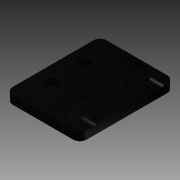
# Autodesk Inventor part: GANTRY SIDE PLATE
Saved by Autodesk Inventor 2013 (Build 170138000, 138)
## iProperties
Created: 2014-03-03
Part Number: GANTRY SIDE PLATE
Material: Generic
Document SubType Name: Modeling
Designer: employee
Density: 1 g/cm^3
Author: employee
Autodesk Inventor part; units mm, degrees
ref_plane "YZ Plane" through (0, 0, 0) normal (1, 0, 0) x (0, 1, 0)
ref_plane "XZ Plane" through (0, 0, 0) normal (0, 1, 0) x (-1, 0, 0)
ref_plane "XY Plane" through (0, 0, 0) normal (0, 0, 1) x (1, 0, 0)
sketch "Sketch1" plane through (0, 0, 0) normal (0, 0, 1) x (1, 0, 0)
  line L0 (0, 35) -> (55, 35)
  line L1 (55, -35) -> (0, -35)
  line L2 (0, -35) -> (0, 35)
  line L3 (11, 12.5) -> (11, -12.5) construction
  circle A0 centre (11, 12.5) radius 11 construction
  circle A1 centre (11, -12.5) radius 11 construction
  circle A2 centre (11, 12.5) radius 4
  circle A3 centre (11, -12.5) radius 4
  line L4 (27.1967, 8.5) -> (37.8033, 8.5) construction
  line L5 (37.8033, 8.5) -> (37.8033, -8.5) construction
  line L6 (37.8033, -8.5) -> (27.1967, -8.5) construction
  line L7 (27.1967, -8.5) -> (27.1967, 8.5) construction
  line L8 (37.8033, 8.5) -> (27.1967, 8.5)
  line L9 (27.1967, 8.5) -> (27.1967, 32.5)
  line L10 (27.1967, 32.5) -> (37.8033, 32.5)
  line L11 (37.8033, 32.5) -> (37.8033, 8.5)
  line L12 (37.8033, -8.5) -> (27.1967, -8.5)
  line L13 (27.1967, -8.5) -> (27.1967, -32.5)
  line L14 (27.1967, -32.5) -> (37.8033, -32.5)
  line L15 (37.8033, -32.5) -> (37.8033, -8.5)
  circle A4 centre (32.5, 8.5) radius 7.5 construction
  line L16 (32.5, 8.5) -> (37.8033, 3.1967) construction
  line L17 (55, 27.8284) -> (45, 27.8284)
  line L18 (45, 27.8284) -> (45, 22.1716)
  line L19 (45, 22.1716) -> (55, 22.1716)
  line L20 (55, -27.8284) -> (45, -27.8284)
  line L21 (45, -27.8284) -> (45, -22.1716)
  line L22 (45, -22.1716) -> (55, -22.1716)
  line L23 (55, -27.8284) -> (55, -35)
  line L24 (55, 35) -> (55, 27.8284)
  line L25 (55, 22.1716) -> (55, -22.1716)
  circle A5 centre (45, 25) radius 4 construction
  line L26 (45, 25) -> (42.1716, 22.1716) construction
  point P0 (0, 0)
  point P1 (0, 0)
  point P2 (11, 0)
  point P3 (27.1967, 0)
  point P4 (45, -25)
  dimension "d7" = 15
  dimension "d16" = 8
  dimension "d0" = 70
  dimension "d2" = 11
  dimension "d3" = 25
  dimension "d4" = 8
  dimension "d5" = 24
  dimension "d6" = 45
  dimension "d9" = 2.5
  dimension "d11" = 22.5
  dimension "d12" = 55
  dimension "d13" = 10
  dimension "d15" = 45
  dimension "d17" = 10
  constraints: 54 end point, 13 parallel, 8 perpendicular, 6 coincident, 6 equal length, 6 horizontal, 6 midpoint, 4 centre point, 3 horizontal alignment, 2 equal radius, 1 point on line, 1 tangent, 6 other
  measures "d0" distance of L1.end L0.start
  measures "d2" distance between parallel lines of L3 L2
  measures "d3" distance of L3.start L3.end
  measures "d4" diameter of A2
  measures "d5" distance of L4.start L9.end
  measures "d6" angle of L8 L16
  measures "d9" distance between parallel lines of L0 L10
  measures "d11" distance from line of L25 L16.start
  measures "d12" distance of L1.start L1.end
  measures "d13" distance from line of L0 point (45, 25)
  measures "d15" angle of L18 L26
  measures "d17" distance of L18.end L19.end
extrude "Extrusion1" add sketch "Sketch1" along normal blind 6.477
sketch "Sketch2" plane through (0, 0, 6.477) normal (0, 0, 1) x (1, 0, 0)
  line L0 (27.1967, 8.5) -> (27.1967, 32.5) projected
  line L1 (27.1967, 32.5) -> (37.8033, 32.5) projected
  line L2 (45, 22.1716) -> (45, 27.8284) projected
  line L3 (45, 27.8284) -> (55, 27.8284) projected
  line L4 (25, 25.5) -> (40, 25.5) construction
  line L5 (40, 25.5) -> (40, 15.5) construction
  line L6 (40, 15.5) -> (25, 15.5) construction
  line L7 (25, 15.5) -> (25, 25.5) construction
  line L8 (48, 29) -> (52, 29) construction
  line L9 (52, 29) -> (52, 21) construction
  line L10 (52, 21) -> (48, 21) construction
  line L11 (48, 21) -> (48, 29) construction
  line L12 (25, 25.5) -> (23.5, 25.5)
  line L13 (23.5, 25.5) -> (23.5, 29.5)
  line L14 (23.5, 29.5) -> (25, 29.5)
  line L15 (25, 29.5) -> (25, 25.5)
  line L16 (40, 25.5) -> (41.5, 25.5)
  line L17 (41.5, 25.5) -> (41.5, 29.5)
  line L18 (41.5, 29.5) -> (40, 29.5)
  line L19 (40, 29.5) -> (40, 25.5)
  line L20 (40, 15.5) -> (41.5, 15.5)
  line L21 (41.5, 15.5) -> (41.5, 11.5)
  line L22 (41.5, 11.5) -> (40, 11.5)
  line L23 (40, 11.5) -> (40, 15.5)
  line L24 (25, 15.5) -> (23.5, 15.5)
  line L25 (23.5, 15.5) -> (23.5, 11.5)
  line L26 (23.5, 11.5) -> (25, 11.5)
  line L27 (25, 11.5) -> (25, 15.5)
  line L28 (48, 21) -> (52, 21)
  line L29 (52, 21) -> (52, 19.5)
  line L30 (52, 19.5) -> (48, 19.5)
  line L31 (48, 19.5) -> (48, 21)
  line L32 (52, 29) -> (48, 29)
  line L33 (48, 29) -> (48, 30.5)
  line L34 (48, 30.5) -> (52, 30.5)
  line L35 (52, 30.5) -> (52, 29)
  point P0 (0, 0)
  point P1 (25, 20.5)
  point P2 (27.1967, 20.5)
  point P3 (48, 25)
  point P4 (45, 25)
  point P5 (50, 29)
  point P6 (50, 27.8284)
  point P7 (32.5, 25.5)
  point P8 (32.5, 32.5)
  point P9 (25, 27.5)
  dimension "d20" = 4
  dimension "d22" = 1.5
  dimension "d23" = 8
  dimension "d24" = 15
  dimension "d25" = 5
  constraints: 64 end point, 16 parallel, 9 equal length, 9 midpoint, 8 horizontal, 8 perpendicular, 2 horizontal alignment, 2 vertical alignment
  measures "d20" distance of L29.end L30.end
  measures "d22" distance of L30.end L10.end
  measures "d23" distance between parallel lines of L8 L28
  measures "d24" distance of L4.start L4.end
  measures "d25" distance from line of L1 point (25, 27.5)
extrude "Extrusion2" cut sketch "Sketch2" against normal through all
mirror "Mirror1" about plane through (0, 0, 0) normal (0, 1, 0) of "Extrusion2"
fillet "Fillet1" radius 5 4 edges at (55, -35, 3.2385) (0, -35, 3.2385) (0, 35, 3.2385) (55, 35, 3.2385)
sketch "Sketch3" plane through (27.1967, 32.5, 0) normal (0, -1, 0) x (1, 0, 0)
  line L0 (10.6066, 0) -> (0, 0) projected
  line L1 (10.6066, 0) -> (10.6066, 6.477) projected
  line L2 (0, 6.477) -> (10.6066, 6.477) projected
  line L3 (0, 0) -> (0, 6.477) projected
  arc A0 (0, 6.477) -> (10.6066, 6.477) centre (5.3033, 11.7803) ccw
  point P0 (-27.1967, 0)
  dimension "d29" = 15
  constraints: 2 end point, 2 point on circle, 1 centre point
  measures "d29" diameter of A0
extrude "Extrusion3" add sketch "Sketch3" along normal up to surface (65 mm away) contours L0 L3 A0 L1
sketch "Sketch4" plane through (45, 22.1716, 0) normal (1, 0, 0) x (0, 0, -1)
  line L0 (0, 5.6569) -> (0, 0) projected
  line L1 (0, 5.6569) -> (-6.477, 5.6569) projected
  line L2 (-6.477, 0) -> (-6.477, 5.6569) projected
  line L3 (0, 0) -> (-6.477, 0) projected
  arc A0 (-6.477, 0) -> (-6.477, 5.6569) centre (-9.3054, 2.8284) ccw
  point P0 (0, -22.1716)
  dimension "d33" = 8
  constraints: 2 end point, 2 point on circle, 1 centre point
  measures "d33" diameter of A0
extrude "Extrusion4" add sketch "Sketch4" along normal up to surface (10 mm away) contours L0 L3 A0 L1
mirror "Mirror2" about plane through (0, 0, 0) normal (0, 1, 0) of "Extrusion4"
body "Solid1"
